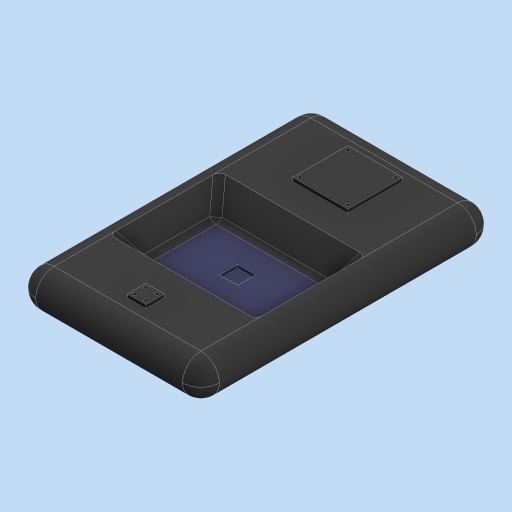
# Autodesk Inventor part: hull
Saved by Autodesk Inventor 2023 (Build 270158000, 158)
## iProperties
Created: 2024-11-14
Part Number: hull
Material: Generic
Document SubType Name: Modeling
Designer: ADMIN
Density: 1 g/cm^3
Appearance: Rubber - Black
Author: ADMIN
Autodesk Inventor part; units mm, degrees
ref_plane "YZ Plane" through (0, 0, 0) normal (1, 0, 0) x (0, 1, 0)
ref_plane "XZ Plane" through (0, 0, 0) normal (0, 1, 0) x (-1, 0, 0)
ref_plane "XY Plane" through (0, 0, 0) normal (0, 0, 1) x (1, 0, 0)
sketch "Sketch1" plane through (0, 0, 0) normal (0, 1, 0) x (-1, 0, 0)
  line L0 (-250, -400) -> (250, -400)
  line L1 (250, -400) -> (250, 400)
  line L2 (250, 400) -> (-250, 400)
  line L3 (-250, 400) -> (-250, -400)
  line L4 (-250, -400) -> (250, 400) construction
  line L5 (250, -400) -> (-250, 400) construction
  point P0 (0, 0)
  point P1 (0, 0)
  dimension "d0" = 800
  dimension "d1" = 500
  constraints: 12 end point, 2 midpoint, 2 parallel, 1 coincident, 1 horizontal, 1 perpendicular
  measures "d0" distance of L0.end L1.end
  measures "d1" distance of L1.end L2.end
extrude "Extrusion1" add sketch "Sketch1" along normal blind 100
fillet "Fillet1" radius 50 12 edges at (250, 100, 0) (250, 0, 0) (0, 100, 400) (0, 0, 400) (-250, 100, 0) (0, 100, -400) (-250, 0, 0) (0, 0, -400) (250, 50, -400) (-250, 50, -400) (-250, 50, 400) (250, 50, 400)
ref_plane "Work Plane1" through (0, 30, 0) normal (0, -1, 0) x (1, 0, 0)
sketch "Sketch6" plane through (0, 100, 0) normal (0, 1, 0) x (1, 0, 0)
  line L0 (200, -200) -> (-200, -200)
  line L1 (-200, -200) -> (-200, 100)
  line L2 (-200, 100) -> (200, 100)
  line L3 (200, 100) -> (200, -200)
  line L4 (200, -200) -> (-200, 100) construction
  line L5 (-200, -200) -> (200, 100) construction
  point P0 (0, -50)
  point P1 (0, 0)
  dimension "d16" = 400
  dimension "d17" = 300
  dimension "d25" = 50
  constraints: 12 end point, 2 midpoint, 2 parallel, 1 horizontal, 1 perpendicular
  measures "d16" distance of L1.end L2.end
  measures "d17" distance of L0.end L1.end
  measures "d25" distance of point (0, 0) point (0, -50)
sketch "Sketch7" plane through (0, 30, 0) normal (0, -1, 0) x (1, 0, 0)
  line L0 (160, 150) -> (-160, 150)
  line L1 (-160, 150) -> (-160, -50)
  line L2 (-160, -50) -> (160, -50)
  line L3 (160, -50) -> (160, 150)
  line L4 (160, 150) -> (-160, -50) construction
  line L5 (-160, 150) -> (160, -50) construction
  line L6 (0, -610.4339) -> (0, 862.6035) projected
  point P0 (0, 50)
  point P1 (0, 0)
  dimension "d18" = 200
  dimension "d27" = 320
  dimension "d28" = 50
  constraints: 12 end point, 2 midpoint, 2 parallel, 1 horizontal, 1 perpendicular, 1 point on line
  measures "d18" distance of L0.end L1.end
  measures "d27" distance of L1.end L2.end
  measures "d28" distance of point (0, 0) point (0, 50)
loft "Loft1" cut profiles "Sketch7", "Sketch6"
fillet "Fillet2" radius 20 8 edges at (-160, 30, 50) (0, 30, -50) (160, 30, 50) (0, 30, 150) (-180, 65, 175) (-180, 65, -75) (180, 65, -75) (180, 65, 175)
sketch "Sketch8" plane through (0, 100, 0) normal (0, 1, 0) x (1, 0, 0)
  line L0 (75, 175) -> (-75, 175)
  line L1 (-75, 175) -> (-75, 325)
  line L2 (-75, 325) -> (75, 325)
  line L3 (75, 325) -> (75, 175)
  line L4 (75, 175) -> (-75, 325) construction
  line L5 (-75, 175) -> (75, 325) construction
  line L6 (0, 560) -> (0, -560) projected
  line L7 (-200, 350) -> (200, 350) projected
  line L8 (25, -325) -> (-25, -325)
  line L9 (-25, -325) -> (-25, -275)
  line L10 (-25, -275) -> (25, -275)
  line L11 (25, -275) -> (25, -325)
  line L12 (25, -325) -> (-25, -275) construction
  line L13 (-25, -325) -> (25, -275) construction
  circle A0 centre (-15, -285) radius 5
  line L14 (200, -350) -> (-200, -350) projected
  circle A1 centre (15, -285) radius 5
  circle A2 centre (-15, -315) radius 5
  circle A3 centre (15, -315) radius 5
  point P0 (0, 0)
  point P1 (0, 250)
  point P2 (0, 350)
  point P3 (0, -300)
  dimension "d30" = 150
  dimension "d31" = 150
  dimension "d32" = 100
  dimension "d67" = 50
  dimension "d68" = 50
  dimension "d71" = 10
  dimension "d72" = 10
  dimension "d73" = 50
  dimension "d76" = 30
  dimension "d79" = 30
  constraints: 24 end point, 5 midpoint, 4 centre point, 4 parallel, 3 horizontal, 3 point on line, 2 perpendicular, 1 vertical, 6 other
  measures "d30" distance of L0.end L1.end
  measures "d31" distance of L1.end L2.end
  measures "d32" distance of point (0, 350) point (0, 250)
  measures "d67" distance of L8.end L9.end
  measures "d68" distance of L8.start L8.end
  measures "d71" diameter of A0
  measures "d72" distance from line of L10 A0.centre
  measures "d73" distance from line of L14 point (0, -300)
  measures "d76" distance of A0.centre A1.centre
  measures "d79" distance of A0.centre A2.centre
extrude "Extrusion2" add sketch "Sketch8" along normal blind 10
sketch "Sketch10" plane through (0, 110, 0) normal (0, 1, 0) x (1, 0, 0)
  circle A0 centre (-65, 315) radius 5
  line L0 (75, 325) -> (-75, 325) projected
  line L1 (-75, 325) -> (-75, 175) projected
  circle A1 centre (65, 315) radius 5
  circle A2 centre (-65, 185) radius 5
  circle A3 centre (65, 185) radius 5
  point P0 (0, 0)
  dimension "d35" = 10
  dimension "d36" = 10
  dimension "d37" = 10
  dimension "d40" = 130
  dimension "d43" = 130
  constraints: 4 centre point, 1 horizontal, 1 vertical, 6 other
  measures "d35" distance from line of L0 A0.centre
  measures "d36" diameter of A0
  measures "d37" distance from line of L1 A0.centre
  measures "d40" distance of A0.centre A1.centre
  measures "d43" distance of A0.centre A2.centre
hole "Hole1" at (-65, 110, -315) at (-65, 110, -185) at (65, 110, -185) at (65, 110, -315) direction (0, -1, 0) diameter 10 depth 10 tip angle 118
thread "Thread1" size "M10x1.5" class "6H" standard "ANSI Metric M Profile" length 8
thread "Thread2" size "M10x1.5" class "6H" standard "ANSI Metric M Profile" length 8
thread "Thread3" size "M10x1.5" class "6H" standard "ANSI Metric M Profile" length 8
thread "Thread4" size "M10x1.5" class "6H" standard "ANSI Metric M Profile" length 8
sketch "Sketch11" plane through (-148.3935, 30, -39.7076) normal (0, 1, 0) x (1, 0, 0)
  line L0 (173.3935, -114.7076) -> (123.3935, -114.7076)
  line L1 (123.3935, -114.7076) -> (123.3935, -64.7076)
  line L2 (123.3935, -64.7076) -> (173.3935, -64.7076)
  line L3 (173.3935, -64.7076) -> (173.3935, -114.7076)
  line L4 (173.3935, -114.7076) -> (123.3935, -64.7076) construction
  line L5 (123.3935, -114.7076) -> (173.3935, -64.7076) construction
  line L6 (148.3935, 520.2924) -> (148.3935, -599.7076) projected
  line L7 (296.7871, -179.4153) -> (0, -179.4153) projected
  line L8 (0, 0) -> (296.7871, 0) projected
  point P0 (148.3935, -39.7076)
  point P1 (148.3935, -89.7076)
  dimension "d61" = 50
  dimension "d62" = 50
  dimension "d63" = 179.4153
  dimension "d64" = 89.7076
  constraints: 12 end point, 2 midpoint, 2 parallel, 1 horizontal, 1 perpendicular, 1 point on line
  measures "d61" distance of L0.end L1.end
  measures "d62" distance of L1.end L2.end
  measures "d63" distance between parallel lines of L7 L8
  measures "d64" distance from line of L8 point (148.394, -89.708)
extrude "Extrusion3" cut sketch "Sketch11" against normal blind 10
extrude "Extrusion4" add sketch "Sketch8" along normal blind 10 contours L10 L11 L8 L6 | L6 L8 L9 L10 | A0 | A1 | A2 | A3
sketch "Sketch12" plane through (0, 110, 0) normal (0, 1, 0) x (1, 0, 0)
  circle A0 centre (-15, -285) radius 5
  line L0 (25, -275) -> (-25, -275) projected
  line L1 (-25, -275) -> (-25, -325) projected
  circle A1 centre (15, -285) radius 5
  circle A2 centre (-15, -315) radius 5
  circle A3 centre (15, -315) radius 5
  point P0 (0, 0)
  dimension "d82" = 10
  dimension "d83" = 10
  dimension "d84" = 10
  dimension "d87" = 30
  dimension "d90" = 30
  constraints: 4 centre point, 1 horizontal, 1 vertical, 6 other
  measures "d82" distance from line of L0 A0.centre
  measures "d83" distance from line of L1 A0.centre
  measures "d84" diameter of A0
  measures "d87" distance of A0.centre A1.centre
  measures "d90" distance of A0.centre A2.centre
hole "Hole2" at (-15, 110, 315) at (-15, 110, 285) at (15, 110, 285) at (15, 110, 315) direction (0, -1, 0) diameter 10 depth 10 tip angle 118
thread "Thread5" size "M10x1.5" class "6H" standard "ANSI Metric M Profile" length 8
thread "Thread6" size "M10x1.5" class "6H" standard "ANSI Metric M Profile" length 8
thread "Thread7" size "M10x1.5" class "6H" standard "ANSI Metric M Profile" length 8
thread "Thread8" size "M10x1.5" class "6H" standard "ANSI Metric M Profile" length 8
sketch "Sketch13" plane through (0, 0, 0) normal (0, -1, 0) x (1, 0, 0)
  line L0 (-137.3, -315.8877) -> (-162.7, -315.8877)
  line L1 (-162.7, -315.8877) -> (-162.7, -284.1123)
  line L2 (-162.7, -284.1123) -> (-137.3, -284.1123)
  line L3 (-137.3, -284.1123) -> (-137.3, -315.8877)
  line L4 (-137.3, -315.8877) -> (-162.7, -284.1123) construction
  line L5 (-162.7, -315.8877) -> (-137.3, -284.1123) construction
  line L6 (-200, -350) -> (-200, 350) projected
  line L7 (200, -350) -> (-200, -350) projected
  line L8 (0, 0) -> (0, -457.6258) construction
  line L9 (137.3, -315.8877) -> (162.7, -315.8877)
  line L10 (162.7, -315.8877) -> (162.7, -284.1123)
  line L11 (162.7, -284.1123) -> (137.3, -284.1123)
  line L12 (137.3, -284.1123) -> (137.3, -315.8877)
  line L13 (137.3, -315.8877) -> (162.7, -284.1123) construction
  line L14 (162.7, -315.8877) -> (137.3, -284.1123) construction
  circle A0 centre (-157.0104, -300) radius 1.7526
  circle A1 centre (-142.9896, -300) radius 1.7526
  line L15 (137.3, -315.8877) -> (162.7, -315.8877)
  circle A2 centre (157.0104, -300) radius 1.7526
  circle A3 centre (142.9896, -300) radius 1.7526
  point P0 (-150, -300)
  point P1 (150, -300)
  dimension "d108" = 31.7754
  dimension "d109" = 25.4
  dimension "d110" = 50
  dimension "d111" = 50
  dimension "d112" = 3.5052
  dimension "d113" = 3.5052
  dimension "d114" = 5.6896
  dimension "d115" = 5.6896
  dimension "d116" = 15.8877
  dimension "d117" = 15.8877
  constraints: 28 end point, 7 symmetric about line, 4 centre point, 2 midpoint, 2 parallel, 1 horizontal, 1 perpendicular, 1 vertical, 2 other
  measures "d108" distance of L0.end L1.end
  measures "d109" distance of L1.end L2.end
  measures "d110" distance from line of L6 point (-150, -300)
  measures "d111" distance from line of L7 point (-150, -300)
  measures "d112" diameter of A0
  measures "d113" diameter of A1
  measures "d114" distance from line of L1 A0.centre
  measures "d115" distance from line of L3 A1.centre
  measures "d116" distance from line of L0 A0.centre
  measures "d117" distance from line of L0 A1.centre
extrude "Extrusion5" add sketch "Sketch13" along normal blind 10
sketch "Sketch15" plane through (137.3, 0, -284.1123) normal (0, 0, 1) x (1, 0, 0)
  circle A0 centre (12.7, 62.8148) radius 73.914
  circle A1 centre (-287.3, 62.8148) radius 73.914
  line L0 (25.4, -10) -> (0, -10) projected
  line L1 (-274.6, -10) -> (-300, -10) projected
  point P0 (-137.3, 0)
  dimension "d124" = 147.828
  dimension "d125" = 147.828
  constraints: 4 point on circle, 2 centre point
  measures "d124" diameter of A0
  measures "d125" diameter of A1
extrude "Extrusion7" add sketch "Sketch15" against normal up to surface (31.7754 mm away) contours L0 A0 | L1 A1 picked at (11.2826, -10.3256) picked at (-288.7174, -10.3256)
extrude "Extrusion8" cut sketch "Sketch13" along normal through all contours A0 | A1 | A2 | A3
equation "\"d28\" = d25"
equation "\"d64\" = 0.5 * d63"
equation "\"d83\" = d82"
equation "\"d84\" = d82"
equation "\"d113\" = d112"
equation "\"d125\" = d124"
body "Solid1"
